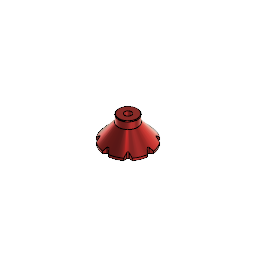
Bed Thumb Screw (Autodesk Fusion 360 design; units mm, degrees)
Autodesk Fusion 360 part; units mm, degrees
sketch "Sketch1" plane through (0, 0, 14) normal (0, 0, 1) x (-1, 0, 0)
  circle A0 centre (-10, -32) radius 2.75
  circle A1 centre (-10, -32) radius 19
  circle A2 centre (-10, -32) radius 6.5
  circle A3 centre (-10, -32) radius 7 construction
  circle A4 centre (-10, -32) radius 13 construction
  point P0 (-10, -32)
  dimension "d741" = 38
  dimension "d747" = 0.5
  dimension "d793" = 0
  dimension "d794" = 0
  dimension "d795" = 0
  dimension "d796" = 0
  dimension "d809" = 0
  dimension "d810" = 0
  dimension "d811" = 0
  dimension "d812" = 0
  dimension "d893" = 0
  dimension "d894" = 0
  dimension "d895" = 0
  dimension "d896" = 0
  dimension "d978" = 13.5
  dimension "d980" = 14
  dimension "d992" = 0
  dimension "d993" = 0
  dimension "d994" = 0
  dimension "d995" = 0
  dimension "d1016" = 26
  dimension "d1018" = 0
  dimension "d1019" = 0
  dimension "d1020" = 0
  dimension "d1021" = 0
  dimension "d1053" = 0
  dimension "d1054" = 0
  dimension "d1055" = 0
  dimension "d1056" = 0
  dimension "d1065" = 0
  dimension "d1066" = 0
  dimension "d1067" = 0
  dimension "d1068" = 0
  dimension "d1368" = 0
  dimension "d1369" = 0
  dimension "d1370" = 0
  dimension "d1371" = 0
  constraint coincident P0 A0.centre
  constraint concentric A0 A4
  constraint concentric A1 A4
  measures "d741" diameter of A1
  measures "d747" distance of A2 A3
  measures "d980" diameter of A3
  measures "d1016" diameter of A4
extrude "Extrude1" add sketch "Sketch1" against normal blind 7 contours A2
sketch "Sketch2" plane through (0, 0, 7) normal (0, 0, -1) x (1, 0, 0)
  circle A0 centre (10, -32) radius 2.75 construction
  circle A1 centre (10, -32) radius 6.5
  line L0 (14, -34.3094) -> (14, -29.6906)
  line L1 (14, -29.6906) -> (10, -27.3812)
  line L2 (10, -27.3812) -> (6, -29.6906)
  line L3 (6, -29.6906) -> (6, -34.3094)
  line L4 (6, -34.3094) -> (10, -36.6188)
  line L5 (10, -36.6188) -> (14, -34.3094)
  point P0 (10, -32)
  dimension "d781" = 8
  constraint coincident P0 A0.centre
  constraint vertical L0
  measures "d781" distance of L1 L4
extrude "Extrude9" cut sketch "Sketch2" against normal blind 4 contours L0 L1 L2 L3 L4 L5
extrude "Extrude2" add sketch "Sketch1" along normal blind 8 contours A1 | A2
sketch "Sketch7" plane through (0, 0, 14) normal (0, 0, -1) x (1, 0, 0)
  circle A0 centre (10, -32) radius 19
  circle A1 centre (10, -32) radius 12
  dimension "d1360" = 24
  constraint concentric A0 A1
  measures "d1360" diameter of A1
extrude "Extrude12" add sketch "Sketch7" along normal blind 7
chamfer "Chamfer1" distance 11 angle 50 1 edges at (27.7142, 38.8707, 22) measured on face at (-3.5024, 33.0806, 22)
sketch "Sketch8" plane through (0, 0, 7) normal (0, 0, -1) x (1, 0, 0)
  circle A0 centre (10, -32) radius 19
  circle A1 centre (10, -32) radius 12
  circle A2 centre (10, -32) radius 19
  line L0 (10, -32) -> (10, -13) construction
  line L1 (7.5, -13.1652) -> (10, -16)
  line L2 (12.5, -13.1652) -> (10, -16)
  point P0 (10, -32)
  dimension "d1348" = 38
  dimension "d1352" = 3
  dimension "d1353" = 5
  constraint coincident P0 A0.centre
  constraint coincident A0 L0.end
  constraint vertical L0
  constraint coincident A2 L1.start
  constraint coincident L0 L1.end
  constraint coincident A0 L2.start
  constraint symmetric L0 L1.start L2.start
  measures "d1348" diameter of A0
  measures "d1352" distance of L0.end L1.end
  measures "d1353" distance of L1.start L2.start
extrude "Extrude13" cut sketch "Sketch8" against normal blind 9 contours A0 A2 L1 L2 picked at (10, -14.0123)
fillet "Fillet2" radius 1 1 edges at (10, 16, 9.733)
pattern_circular "C-Pattern2" count 8 over 360 about axis through (10, 32, 7) along (0, 0, -1) of "Extrude13", "Fillet2"
extrude "Extrude10" add 1 faces at (14.8301, 28.0605, 22) along direction (0, 0, 1) blind 6
chamfer "Chamfer4" distance 0.5 angle 45 1 edges at (17.4586, 34.8929, 28)
chamfer "Chamfer5" distance 2 angle 45 1 edges at (-1.1879, 27.6606, 7)
named bodies: "Bed Thumb Screw"
